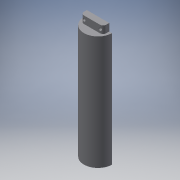
# Autodesk Inventor part: Bottom tube
Saved by Autodesk Inventor 2019 (Build 230136000, 136)
## iProperties
Created: 2018-10-29
Part Number: Bottom tube
Material: Generic
Document SubType Name: Modeling
Designer: Derek Fronek
Density: 1 g/cm^3
Appearance: Default
Author: Derek Fronek
Autodesk Inventor part; units mm, degrees
ref_plane "YZ Plane" through (0, 0, 0) normal (1, 0, 0) x (0, 1, 0)
ref_plane "XZ Plane" through (0, 0, 0) normal (0, 1, 0) x (-1, 0, 0)
sketch "Sketch1" plane through (0, 0, 0) normal (0, 1, 0) x (-1, 0, 0)
  line L0 (-3.9004, 20.5177) -> (-3.9004, 22.0877) projected
  line L1 (-28.9824, 20.5177) -> (-28.9824, 22.0877) projected
  line L2 (-26.4424, 22.0877) -> (-6.4404, 22.0877) projected
  line L3 (-6.4404, 20.5177) -> (-26.4424, 20.5177) projected
  line L4 (-6.36, 29.8752) -> (-26.5228, 29.8752)
  line L5 (-29.6192, 22.5147) -> (-29.6192, 20.0906)
  line L6 (-26.5228, 12.7302) -> (-6.36, 12.7302)
  line L7 (-3.2636, 20.0906) -> (-3.2636, 22.5147)
  line L8 (-3.2636, 29.8752) -> (-29.6192, 12.7302) construction
  line L9 (-29.6192, 29.8752) -> (-3.2636, 12.7302) construction
  circle A0 centre (-16.4414, 21.3027) radius 14.5
  arc A1 (-3.2636, 22.5147) -> (-6.36, 29.8752) centre (-16.4414, 21.3027) ccw
  arc A2 (-26.5228, 29.8752) -> (-29.6192, 22.5147) centre (-16.4414, 21.3027) ccw
  arc A3 (-29.6192, 20.0906) -> (-26.5228, 12.7302) centre (-16.4414, 21.3027) ccw
  arc A4 (-6.36, 12.7302) -> (-3.2636, 20.0906) centre (-16.4414, 21.3027) ccw
  line L10 (-29.6192, 21.3027) -> (-30.9414, 21.3027)
  line L11 (-3.2636, 21.3027) -> (-1.9414, 21.3027)
  point P0 (0, 0)
  dimension "d2" = 17.145
  dimension "d3" = 29
  constraints: 16 end point, 10 point on circle, 5 centre point, 4 midpoint, 2 coincident, 2 horizontal, 2 parallel, 1 perpendicular
  measures "d2" distance of L8.end L9.start
  measures "d3" diameter of A0
extrude "Extrusion1" add sketch "Sketch1" along normal blind 50.8 and the other way blind 63.5 contours L4 A2 L5 L10 A0 L11 L7 A1
sketch "Sketch2" plane through (0, 50.8, 0) normal (0, 1, 0) x (1, 0, 0)
  arc A0 (1.9414, -21.3027) -> (30.9414, -21.3027) centre (16.4414, -21.3027) ccw projected
  line L0 (1.9414, -21.3027) -> (30.9414, -21.3027)
  point P0 (0, 0)
  constraints: 2 end point, 1 horizontal
extrude "Extrusion2" add sketch "Sketch2" along normal blind 3.175
sketch "Sketch4" plane through (29.6192, 50.8, 21.3027) normal (0, 0, -1) x (-1, 0, 0)
  point P0 (29.6192, -50.8)
sketch "Sketch5" plane through (26.5228, -63.5, 29.8752) normal (0, 0, -1) x (-1, 0, 0)
  line L0 (-3.152, 16.0592) -> (3.198, 16.0592)
  line L1 (3.198, 16.0592) -> (3.198, 9.7092)
  line L2 (3.198, 9.7092) -> (-3.152, 9.7092)
  line L3 (23.2592, 16.0592) -> (16.9092, 16.0592)
  line L4 (16.9092, 16.0592) -> (16.9092, 9.7092)
  line L5 (16.9092, 9.7092) -> (23.2592, 9.7092)
  circle A0 centre (0.0804, 13.2129) radius 1.6 projected
  circle A1 centre (20.0824, 13.2129) radius 1.6 projected
  line L6 (-3.152, 16.0592) -> (-3.152, 9.7092)
  line L7 (0, 0) -> (0, 114.3) projected
  line L8 (23.2592, 16.0592) -> (23.2592, 9.7092)
  line L9 (23.2592, 0) -> (23.2592, 114.3) projected
  point P0 (26.5228, 63.5)
  dimension "d13" = 6.35
  dimension "d14" = 6.35
  dimension "d15" = 6.35
  constraints: 16 end point, 3 parallel, 2 horizontal, 2 perpendicular, 1 collinear
  measures "d13" distance of L1.end L2.end
  measures "d14" distance of L0.end L1.end
  measures "d15" distance of L5.end L4.end
extrude "Extrusion4" add sketch "Sketch5" along normal blind 7.62 contours L0 L7 A0 L2 L6 | L0 L1 L2 L7 A0 | L7 A0 | A0 L7 | L8 L5 L4 L3 | A1
sketch "Sketch6" plane through (28.1359, -53.7908, 29.8752) normal (0, -1, 0) x (1, 0, 0)
  line L0 (-23.3891, 0) -> (-24.8723, 0) projected
  line L1 (-24.8723, 0) -> (-24.8723, -2.523) projected
  arc A0 (-23.3891, 0) -> (-24.8723, -2.523) centre (-11.6945, -8.5725) ccw projected
  line L2 (-23.3891, 0) -> (-24.8723, 0) projected
  line L3 (-24.8723, 0) -> (-24.8723, -2.523) projected
  line L4 (0, 0) -> (1.5389, 0) projected
  line L5 (1.5389, 0) -> (1.5389, -2.6457) projected
  arc A1 (1.5389, -2.6457) -> (0, 0) centre (-11.6945, -8.5725) ccw projected
  line L6 (1.5389, 0) -> (1.5389, -2.6457) projected
  line L7 (0, 0) -> (1.5389, 0) projected
  point P0 (-28.1359, -29.8752)
extrude "Extrusion5" cut sketch "Sketch6" against normal blind 7.62
sketch "Sketch7" plane through (26.5228, -63.5, 22.2552) normal (0, 0, -1) x (-1, 0, 0)
  line L0 (20.1628, 0) -> (20.1628, 114.3) projected
  line L1 (20.1628, 18.9379) -> (20.1628, 24.9499) projected
  line L2 (20.1628, 16.0592) -> (20.1628, 9.7092) projected
  circle A0 centre (0.0804, 13.2129) radius 1.6 projected
  circle A1 centre (20.0824, 13.2129) radius 1.6 projected
  point P0 (26.5228, 63.5)
extrude "Extrusion6" cut sketch "Sketch7" against normal blind 5.08
sketch "Sketch8" plane through (26.5228, -63.5, 29.8752) normal (0, 0, -1) x (-1, 0, 0)
  line L0 (20.0824, 110.6729) -> (0.0804, 110.6729) projected
  line L1 (-3.0964, 0) -> (-3.0964, 114.3) projected
  line L2 (-3.0964, 110.6729) -> (3.2536, 110.6729)
  line L3 (3.2536, 110.6729) -> (3.2536, 104.3229)
  line L4 (3.2536, 104.3229) -> (-3.0964, 104.3229)
  line L5 (-3.0964, 104.3229) -> (-3.0964, 110.6729)
  line L6 (23.3057, 110.6729) -> (16.944, 110.6729)
  line L7 (16.944, 110.6729) -> (16.944, 104.3229)
  line L8 (16.944, 104.3229) -> (23.3057, 104.3229)
  line L9 (23.3057, 104.3229) -> (23.3057, 110.6729)
  point P0 (26.5228, 63.5)
  dimension "d22" = 6.35
  dimension "d23" = 6.35
  constraints: 16 end point, 4 parallel, 3 point on line, 2 horizontal, 2 perpendicular
  measures "d22" distance of L3.end L4.end
  measures "d23" distance of L2.end L3.end
extrude "Extrusion7" add sketch "Sketch8" along normal blind 7.62
sketch "Sketch9" plane through (26.5228, -63.5, 22.2552) normal (0, 0, -1) x (-1, 0, 0)
  circle A0 centre (20.0824, 107.8279) radius 1.6 projected
  circle A1 centre (0.0804, 107.8279) radius 1.6 projected
  point P0 (26.5228, 63.5)
extrude "Extrusion8" cut sketch "Sketch9" against normal blind 5.08
sketch "Sketch10" plane through (28.1359, 47.1729, 29.8752) normal (0, 1, 0) x (1, 0, 0)
  arc A0 (-24.9189, 2.6254) -> (-23.3891, 0) centre (-11.6945, 8.5725) ccw projected
  line L0 (-24.9189, 0) -> (-24.9189, 2.6254) projected
  line L1 (-24.9189, 0) -> (-23.3891, 0) projected
  arc A1 (0, 0) -> (1.4832, 2.523) centre (-11.6945, 8.5725) ccw projected
  line L2 (1.4832, 0) -> (0, 0) projected
  line L3 (1.4832, 0) -> (1.4832, 2.523) projected
  point P0 (-28.1359, 29.8752)
extrude "Extrusion9" cut sketch "Sketch10" against normal blind 6.35
sketch "Sketch11" plane through (0, 53.975, 0) normal (0, 1, 0) x (1, 0, 0)
  line L0 (5.0114, -21.3027) -> (28.0517, -21.3027) projected
  line L1 (28.0517, -21.3027) -> (28.0517, -18.1277) projected
  arc A0 (28.0517, -18.1277) -> (24.8767, -14.9527) centre (24.8767, -18.1277) ccw projected
  line L2 (24.8767, -14.9527) -> (8.1864, -14.9527) projected
  arc A1 (8.1864, -14.9527) -> (5.0114, -18.1277) centre (8.1864, -18.1277) ccw projected
  line L3 (5.0114, -18.1277) -> (5.0114, -21.3027) projected
  line L4 (5.0114, -21.3027) -> (28.0517, -21.3027)
  line L5 (28.0517, -21.3027) -> (28.0517, -24.4777)
  line L6 (24.8767, -27.6527) -> (8.1864, -27.6527)
  line L7 (5.0114, -24.4777) -> (5.0114, -21.3027)
  arc A2 (24.8767, -27.6527) -> (28.0517, -24.4777) centre (24.8767, -24.4777) ccw
  arc A3 (5.0114, -24.4777) -> (8.1864, -27.6527) centre (8.1864, -24.4777) ccw
  point P0 (0, 0)
  point P1 (28.0517, -27.6527)
  dimension "d30" = 6.35
  dimension "d31" = 3.175
  constraints: 8 end point, 4 point on circle, 4 tangent, 2 centre point, 2 parallel, 2 point on line, 1 equal radius, 1 horizontal, 1 perpendicular
  measures "d30" distance of L4.end point (28.052, -27.653)
  measures "d31" radius of A2
ref_plane "Work Plane1" through (5.0114, 61.595, 14.9527) normal (0, 1, 0) x (0, 0, 1)
extrude "Extrusion10" add sketch "Sketch11" along normal up to surface (7.62 mm away) contours L0 L5 A2 L6 A3 L7
sketch "Sketch12" plane through (8.1864, 53.975, 27.6527) normal (0, 0, 1) x (1, 0, 0)
  arc A0 (16.6904, 5.3975) -> (16.6904, 2.2225) centre (16.6904, 3.81) ccw
  arc A1 (0, 2.2225) -> (0, 5.3975) centre (0, 3.81) ccw
  spline S0 degree 3 poles (0, 5.3975) (-0.2031, 5.3975) (-0.4174, 5.3562) (-0.8076, 5.193) (-0.9838, 5.0713) (-1.2617, 4.7934) (-1.3831, 4.6174) (-1.546, 4.2277) (-1.5875, 4.0137) (-1.5875, 3.81) (-1.5875, 3.6063) (-1.546, 3.3923) (-1.3831, 3.0026) (-1.2617, 2.8266) (-0.9838, 2.5487) (-0.8076, 2.427) (-0.4174, 2.2638) (-0.2031, 2.2225) (0, 2.2225) knots 0 0 0 0 0.124829 0.124829 0.249659 0.249659 0.374829 0.374829 0.5 0.5 0.5 0.625171 0.625171 0.750341 0.750341 0.875171 0.875171 1 1 1 1
  circle A2 centre (16.6904, 3.81) radius 1.5875
  point P0 (-8.1864, -53.975)
extrude "Extrusion11" cut sketch "Sketch12" against normal blind 7.62
sketch "Sketch13" plane through (26.5228, -63.5, 29.8752) normal (0, 0, -1) x (-1, 0, 0)
  line L0 (-0.6179, 23.6999) -> (-0.6179, 24.9499) projected
  line L1 (2.0488, 20.1879) -> (2.0488, 18.9379) projected
  line L2 (-0.6179, 24.9499) -> (2.0488, 24.9499)
  line L3 (2.0488, 24.9499) -> (2.0488, 18.9379)
  line L4 (2.0488, 18.9379) -> (-0.6179, 18.9379)
  line L5 (-0.6179, 18.9379) -> (-0.6179, 24.9499)
  point P0 (26.5228, 63.5)
  constraints: 8 end point, 2 parallel, 1 horizontal, 1 perpendicular
extrude "Extrusion12" cut sketch "Sketch13" against normal blind 25.4
fillet "Fillet1" radius 3.175 1 edges at (16.4414, 53.975, 35.8027)
body "Solid1"
